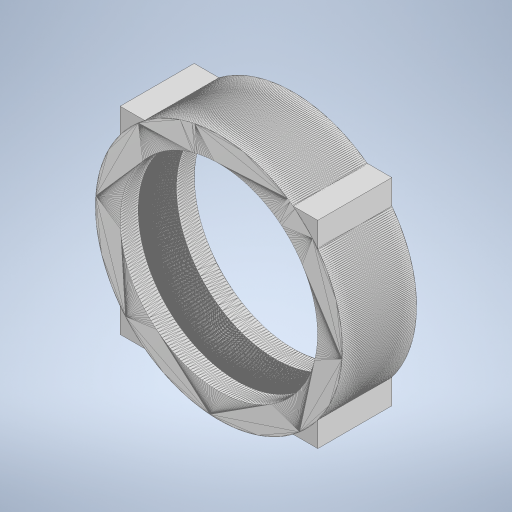
# Autodesk Inventor part: bearing-gairin
Saved by Autodesk Inventor 2024 (Build 280153000, 153)
## iProperties
Created: 2024-02-10
Part Number: bearing-gairin
Material: 一般
Document SubType Name: Modeling
Designer: mott1
Density: 1 g/cm^3
Appearance: 既定
Author: mott1
Autodesk Inventor part; units mm, degrees
ref_plane "YZ Plane" through (0, 0, 0) normal (1, 0, 0) x (0, 1, 0)
ref_plane "XZ Plane" through (0, 0, 0) normal (0, 1, 0) x (-1, 0, 0)
ref_plane "XY Plane" through (0, 0, 0) normal (0, 0, 1) x (1, 0, 0)
sketch "スケッチ1" plane through (8.3334, 12.4721, 4.5) normal (0, 0, 1) x (1, 0, 0)
  circle A0 centre (-8.3334, -12.4721) radius 15
  line L0 (-8.3334, -12.4721) -> (-8.3334, -0.4721)
  line L1 (0.6666, -0.4721) -> (3.6666, -0.4721)
  line L2 (3.6666, -0.4721) -> (-8.3334, -0.4721)
  line L3 (-17.3334, -0.4721) -> (-20.3334, -0.4721)
  line L4 (3.6666, -24.4721) -> (3.6666, -21.4721)
  line L5 (3.6666, -3.4721) -> (3.6666, -0.4721)
  line L6 (-20.3334, -24.4721) -> (-17.3334, -24.4721)
  line L7 (0.6666, -24.4721) -> (3.6666, -24.4721)
  line L8 (-20.3334, -0.4721) -> (-20.3334, -3.4721)
  line L9 (-20.3334, -21.4721) -> (-20.3334, -24.4721)
  dimension "d4" = 30
  dimension "d7" = 12
  dimension "d8" = 12
  dimension "d9" = 24
  dimension "d10" = 24
  constraints: 20 end point, 8 parallel, 5 perpendicular, 2 horizontal, 1 coincident, 1 vertical, 10 other
  measures "d7" distance of L0.start L0.end
  measures "d8" distance of L0.end L1.end
  measures "d9" distance of L4.start L6.start
  measures "d10" distance of L6.start L3.end
extrude "押し出し2" add sketch "スケッチ1" against normal blind 9 contours A0 L1 L5 | L4 L7 A0 | A0 L8 L3 | L6 L9 A0
